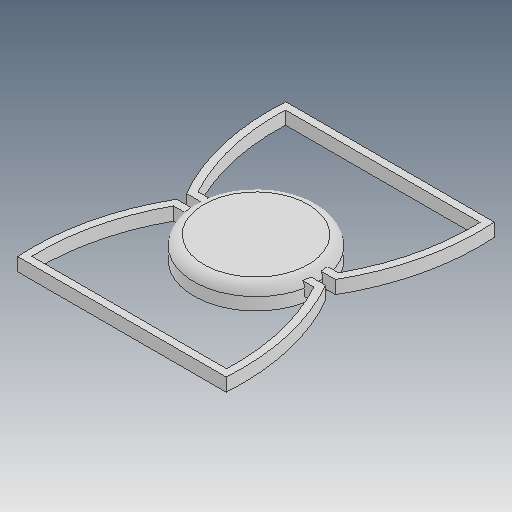
# Autodesk Inventor part: brace_tabs
Saved by Autodesk Inventor 2025.2 (Build 292293000, 293)
## iProperties
Created: 2025-02-17
Part Number: brace_tabs
Material: Generic
Document SubType Name: Modeling
Designer: email
Density: 1 g/cm^3
Appearance: Default
Author: email
Autodesk Inventor part; units mm, degrees
ref_plane "YZ Plane" through (0, 0, 0) normal (1, 0, 0) x (0, 1, 0)
ref_plane "XY Plane" through (0, 0, 0) normal (0, 0, 1) x (1, 0, 0)
sketch "Sketch1" plane through (0, 0, 0) normal (0, 1, 0) x (-1, 0, 0)
  circle A0 centre (0, 0) radius 12.5
  dimension "d0" = 25
  constraints: 1 centre point, 1 coincident
  measures "d0" diameter of A0
extrude "Extrusion1" add sketch "Sketch1" along normal blind 4.5
ref_plane "Work Plane1" through (0, 1, 0) normal (0, 1, 0) x (-1, 0, 0)
sketch "Sketch2" plane through (0, 1, 0) normal (0, 1, 0) x (-1, 0, 0)
  line L0 (15, -1) -> (-15, -1)
  arc A0 (21, -27) -> (15, -1) centre (-24.8954, -23.8989) ccw
  line L1 (21, -27) -> (-21, -27)
  arc A1 (-15, -1) -> (-21, -27) centre (24.8954, -23.8989) ccw
  line L2 (-19.6045, -25.5298) -> (19.6045, -25.5298)
  arc A2 (19.6045, -25.5298) -> (14.1394, -2.4702) centre (-24.8954, -23.8989) ccw
  line L3 (14.1394, -2.4702) -> (-14.1394, -2.4702)
  arc A3 (-14.1394, -2.4702) -> (-19.6045, -25.5298) centre (24.8954, -23.8989) ccw
  line L4 (31.9342, 0) -> (-23.3502, 0) construction
  line L5 (15, 1) -> (-15, 1)
  arc A4 (15, 1) -> (21, 27) centre (-24.8954, 23.8989) ccw
  line L6 (21, 27) -> (-21, 27)
  arc A5 (-21, 27) -> (-15, 1) centre (24.8954, 23.8989) ccw
  line L7 (-19.6045, 25.5298) -> (19.6045, 25.5298)
  arc A6 (14.1394, 2.4702) -> (19.6045, 25.5298) centre (-24.8954, 23.8989) ccw
  line L8 (14.1394, 2.4702) -> (-14.1394, 2.4702)
  arc A7 (-19.6045, 25.5298) -> (-14.1394, 2.4702) centre (24.8954, 23.8989) ccw
  point P0 (0, 0)
  point P1 (0, -1)
  point P2 (0, -27)
  point P3 (0, 1)
  point P4 (0, 27)
  dimension "d4" = 1
  dimension "d5" = 30
  dimension "d6" = 26
  dimension "d7" = 42
  dimension "d8" = 46
  dimension "d9" = 46
  constraints: 18 end point, 16 point on circle, 12 symmetric about line, 8 centre point, 3 horizontal, 2 midpoint, 2 vertical alignment, 7 other
  measures "d4" distance from line of point (0, 0) L0
  measures "d5" distance of L0.start L0.end
  measures "d6" vertical distance of L1.start L0.start
  measures "d7" distance of L1.start L1.end
  measures "d8" radius of A0
  measures "d9" radius of A1
extrude "Extrusion2" add sketch "Sketch2" along normal blind 2.65
fillet "Fillet1" radius 2 1 edges at (12.5, 4.5, 0)
sketch "Sketch3" plane through (0, 0, 0) normal (0, -1, 0) x (1, 0, 0)
  line L0 (-7.886, 0) -> (-6.3799, 4.6353)
  line L1 (-6.3799, 4.6353) -> (-2.4369, 7.5)
  line L2 (-2.4369, 7.5) -> (2.4369, 7.5)
  line L3 (2.4369, 7.5) -> (6.3799, 4.6353)
  line L4 (6.3799, 4.6353) -> (7.886, 0)
  line L5 (7.886, 0) -> (6.3799, -4.6353)
  line L6 (6.3799, -4.6353) -> (2.4369, -7.5)
  line L7 (2.4369, -7.5) -> (-2.4369, -7.5)
  line L8 (-2.4369, -7.5) -> (-6.3799, -4.6353)
  line L9 (-6.3799, -4.6353) -> (-7.886, 0)
  point P0 (0, 0)
  point P1 (0, 0)
  point P2 (0, -7.5)
  dimension "d13" = 15
  constraints: 20 end point, 1 coincident, 1 midpoint, 21 other
  measures "d13" distance from line of L2 point (0, -7.5)
extrude "Extrusion3" add sketch "Sketch3" along normal blind 3
body "Solid1"
